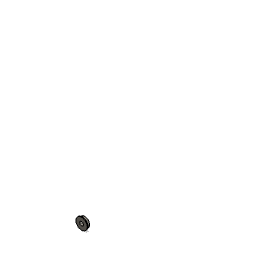
splicer_camera_rgb-filter_bearing-f695 (Autodesk Fusion 360 design; units mm, degrees)
Autodesk Fusion 360 part; units mm, degrees
sketch "Sketch1" plane through (0, 0, 8.7) normal (0, 0, 1) x (1, 0, 0)
  circle A0 centre (46.0559, 45.8678) radius 7.65
  circle A1 centre (46.0559, 45.8678) radius 10
  circle A2 centre (46.0559, 45.8678) radius 7.5
  circle A3 centre (46.0559, 45.8678) radius 6.5
  circle A4 centre (46.0559, 45.8678) radius 2.55
  dimension "d158" = 15
  dimension "d159" = 13
  dimension "d164" = 5.1
  constraint concentric A0 A2
  constraint concentric A2 A3
  constraint concentric A3 A4
  measures "d158" diameter of A2
  measures "d159" diameter of A3
  measures "d164" diameter of A4
extrude "Extrude1" add sketch "Sketch1" against normal blind 4 contours A3 | A4
extrude "Extrude2" add sketch "Sketch1" against normal blind 1 contours A2
extrude "Extrude3" cut sketch "Sketch1" against normal blind 4 contours A4
named bodies: "splicer_camera_rgb-filter_bearing-f695"
